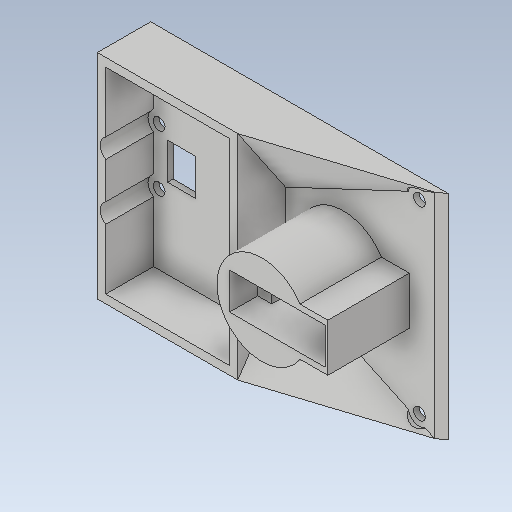
# Autodesk Inventor part: cover
Saved by Autodesk Inventor 2020 (Build 240168000, 168)
## iProperties
Created: 2020-01-29
Part Number: cover
Material: Ogólne
Document SubType Name: Modeling
Designer: blep
Density: 1 g/cm^3
Appearance: Domyślne
Author: blep
Autodesk Inventor part; units mm, degrees
ref_plane "YZ Plane" through (0, 0, 0) normal (1, 0, 0) x (0, 1, 0)
ref_plane "XZ Plane" through (0, 0, 0) normal (0, 1, 0) x (-1, 0, 0)
ref_plane "XY Plane" through (0, 0, 0) normal (0, 0, 1) x (1, 0, 0)
sketch "Sketch1" plane through (0, 0, 0) normal (0, 0, 1) x (1, 0, 0)
  line L0 (47.7059, -35) -> (-50, -35) projected
  line L1 (-50, -35) -> (-50, 35) projected
  line L2 (-50, 35) -> (47.7059, 35) projected
  line L3 (47.7059, 35) -> (47.7059, -35) projected
  line L4 (53, -38) -> (53, 38) projected
  line L5 (53, 38) -> (-53, 38) projected
  line L6 (-53, 38) -> (-53, -38) projected
  line L7 (-53, -38) -> (53, -38) projected
  point P0 (0, 0)
extrude "Extrusion1" add sketch "Sketch1" along normal blind 2 contours L0 L1 L2 L3 | L7 L6 L5 L4
sketch "Sketch2" plane through (-53, 38, 0) normal (0, 1, 0) x (1, 0, 0)
  line L0 (106, 0) -> (130.7184, 17) projected
  line L1 (106, 0) -> (106, -2) projected
  line L2 (106, 0) -> (103.092, -2)
  line L3 (106, -2) -> (0, -2) projected
  line L4 (103.092, -2) -> (106, -2)
  point P0 (53, 0)
  constraints: 4 end point, 1 collinear, 1 point on line
extrude "Extrusion2" cut sketch "Sketch2" against normal through all
sketch "Sketch3" plane through (0, 0, 2) normal (0, 0, 1) x (1, 0, 0)
  line L0 (50.092, -38) -> (50.092, 38) projected
  line L1 (50.092, 38) -> (-53, 38) projected
  line L2 (-53, 38) -> (-53, -38) projected
  line L3 (-53, -38) -> (50.092, -38) projected
  line L4 (-53, -38) -> (-3, -38)
  line L5 (-3, -38) -> (-3, 38)
  line L6 (-3, 38) -> (-53, 38)
  line L7 (-53, 38) -> (-53, -38)
  line L8 (-53, 38) -> (-53, -38) projected
  line L9 (-53, -38) -> (50.092, -38) projected
  line L10 (50.092, 38) -> (-53, 38) projected
  line L11 (-50, -35) -> (-6, -35)
  line L12 (-6, -35) -> (-6, 35)
  line L13 (-6, 35) -> (-50, 35)
  line L14 (-50, 35) -> (-50, -35)
  point P0 (0, 0)
  dimension "d4" = 50
  dimension "d5" = 3
  dimension "d6" = 3
  dimension "d7" = 3
  dimension "d8" = 3
  constraints: 16 end point, 4 parallel, 3 collinear, 2 horizontal, 2 perpendicular
  measures "d4" distance between parallel lines of L2 L5
  measures "d5" distance between parallel lines of L2 L14
  measures "d6" distance between parallel lines of L3 L11
  measures "d7" distance between parallel lines of L1 L13
  measures "d8" distance between parallel lines of L5 L12
extrude "Extrusion3" add sketch "Sketch3" along normal blind 17 contours L3 L2 L1 L5
sketch3d "3D Sketch1"
sketch "Sketch4" plane through (-3, -38, 2) normal (1, 0, 0) x (0, 0, -1)
  line L0 (0, 76) -> (0, 0) projected
  line L1 (0, 76) -> (-17, 76) projected
  line L2 (-17, 0) -> (-17, 76) projected
  line L3 (0, 0) -> (-17, 0) projected
  line L4 (-17, 0) -> (-17, 76) projected
  line L5 (-17, 0) -> (0, 25)
  line L6 (0, 3) -> (0, 73) projected
  line L7 (-17, 76) -> (0, 51)
  point P0 (2, 38)
  dimension "d11" = 25
  dimension "d12" = 25
  constraints: 4 end point, 2 point on line
  measures "d11" distance from line of L3 L5.end
  measures "d12" distance from line of L1 L7.end
loft "Loft1" add profiles "Sketch4" section 2 point at (50.092, -38, 2) contours L5 L0 L3
loft "Loft2" add profiles "Sketch4" section 2 point at (50.092, 38, 2) contours L0 L7 L1
sketch "Sketch6" plane through (0, 0, 2) normal (0, 0, 1) x (1, 0, 0)
  line L0 (11.092, -6.5) -> (35.092, -6.5)
  line L1 (35.092, -6.5) -> (35.092, 6.5)
  line L2 (35.092, 6.5) -> (11.092, 6.5)
  line L3 (11.092, 6.5) -> (11.092, -6.5)
  line L4 (50.092, -38) -> (50.092, 38) construction
  line L5 (50.092, 38) -> (35.092, 6.5) construction
  line L6 (50.092, -38) -> (35.092, -6.5) construction
  line L7 (11.092, -6.5) -> (35.092, 6.5) construction
  line L8 (11.092, 6.5) -> (35.092, -6.5) construction
  line L9 (5.092, -8.5) -> (41.092, -8.5)
  line L10 (41.092, -8.5) -> (41.092, 8.5)
  line L11 (41.092, 8.5) -> (5.092, 8.5)
  line L12 (5.092, 8.5) -> (5.092, -8.5)
  point P0 (0, 0)
  point P1 (23.092, 0)
  dimension "d25" = 24
  dimension "d26" = 13
  dimension "d27" = 15
  dimension "d31" = 6
  dimension "d32" = 6
  dimension "d33" = 2
  dimension "d34" = 2
  constraints: 24 end point, 4 parallel, 2 horizontal, 2 perpendicular, 1 equal length, 1 midpoint
  measures "d25" distance of L2.end L1.end
  measures "d26" distance of L1.end L0.end
  measures "d27" distance between parallel lines of L4 L1
  measures "d31" distance between parallel lines of L12 L3
  measures "d32" distance between parallel lines of L10 L1
  measures "d33" distance between parallel lines of L9 L0
  measures "d34" distance between parallel lines of L11 L2
extrude "Extrusion5" add sketch "Sketch6" along normal blind 19
sketch "Sketch7" plane through (0, 0, 2) normal (0, 0, 1) x (1, 0, 0)
  circle A0 centre (17.592, 0) radius 0.6 projected
  arc A1 (31.1474, 8.5) -> (31.1474, -8.5) centre (17.592, 0) ccw
  line L0 (31.1474, -8.5) -> (5.092, -8.5)
  line L1 (5.092, -8.5) -> (5.092, 8.5)
  line L2 (5.092, 8.5) -> (31.1474, 8.5)
  line L3 (5.092, -8.5) -> (5.092, 8.5) projected
  line L4 (41.092, -8.5) -> (5.092, -8.5) projected
  line L5 (5.092, 8.5) -> (41.092, 8.5) projected
  point P0 (0, 0)
  dimension "d35" = 32
  constraints: 6 end point, 3 collinear, 2 point on circle, 2 point on line, 1 centre point, 1 coincident
  measures "d35" diameter of A1
extrude "Extrusion6" add sketch "Sketch7" along normal blind 19 contours L2 L1 L0 A1
sketch "Sketch8" plane through (0, 0, 21) normal (0, 0, 1) x (1, 0, 0)
  line L0 (6.592, -1.125) -> (6.592, -6.2) projected
  line L1 (6.592, 6.2) -> (6.592, 1.125) projected
  line L2 (11.092, 6.5) -> (35.092, 6.5) projected
  line L3 (35.092, -6.5) -> (11.092, -6.5) projected
  line L4 (39.592, 6.2) -> (39.592, 1.125) projected
  line L5 (39.592, -1.125) -> (39.592, -6.2) projected
  line L6 (6.092, -6.5) -> (40.092, -6.5)
  line L7 (40.092, -6.5) -> (40.092, 6.5)
  line L8 (40.092, 6.5) -> (6.092, 6.5)
  line L9 (6.092, 6.5) -> (6.092, -6.5)
  arc A0 (31.1474, 8.5) -> (31.1474, -8.5) centre (17.592, 0) ccw projected
  line L10 (31.1474, -8.5) -> (41.092, -8.5) projected
  line L11 (41.092, 8.5) -> (31.1474, 8.5) projected
  line L12 (41.092, -8.5) -> (41.092, 8.5) projected
  point P0 (0, 0)
  dimension "d38" = 0.5
  dimension "d39" = 0.5
  constraints: 8 end point, 2 collinear, 2 parallel, 1 horizontal, 1 perpendicular
  measures "d38" distance between parallel lines of L7 L4
  measures "d39" distance between parallel lines of L1 L9
ref_plane "Work Plane1" through (12.092, -5.5, 31) normal (0, 0, 1) x (1, 0, 0)
extrude "Extrusion7" add sketch "Sketch8" along normal up to surface (10 mm away)
sketch "Sketch9" plane through (0, 0, 21) normal (0, 0, 1) x (1, 0, 0)
  arc A0 (8.4305, -0.75) -> (8.4305, 0.75) centre (9.092, 0) ccw projected
  arc A1 (37.7534, 0.75) -> (37.7534, -0.75) centre (37.092, 0) ccw projected
  point P0 (0, 0)
hole "Hole1" at (9.092, 0, 21) at (37.092, 0, 21) direction (0, 0, -1) diameter 1 depth 5 tip angle 118
sketch "Sketch10" plane through (0, 0, 2) normal (0, 0, 1) x (1, 0, 0)
  line L0 (7.592, -4.5) -> (11.092, -4.5)
  line L1 (11.092, -4.5) -> (11.092, 4.5)
  line L2 (11.092, 4.5) -> (7.592, 4.5)
  line L3 (7.592, 4.5) -> (7.592, -4.5)
  line L4 (11.092, 6.5) -> (11.092, -6.5) projected
  line L5 (35.092, 6.5) -> (11.092, 6.5) construction
  line L6 (11.092, 6.5) -> (7.592, 4.5) construction
  line L7 (7.592, -4.5) -> (11.092, -6.5) construction
  point P0 (0, 0)
  dimension "d49" = 3.5
  dimension "d50" = 9
  constraints: 12 end point, 2 parallel, 1 collinear, 1 equal length, 1 horizontal, 1 perpendicular
  measures "d49" distance of L2.end L1.end
  measures "d50" distance of L1.end L0.end
extrude "Extrusion8" cut sketch "Sketch10" along normal blind 14 and the other way blind 3
sketch "Sketch11" plane through (0, 0, 0) normal (0, 0, -1) x (-1, 0, 0)
  circle A0 centre (-44.7059, -33) radius 2.125 projected
  circle A1 centre (-44.7059, 33) radius 2.125 projected
  circle A2 centre (48, -10) radius 2.125 projected
  circle A3 centre (48, 10) radius 2.125 projected
  point P0 (0, 0)
extrude "Extrusion9" cut sketch "Sketch11" against normal through all
sketch "Sketch12" plane through (0, 0, 2) normal (0, 0, 1) x (1, 0, 0)
  circle A0 centre (44.7059, -33) radius 2.125 projected
  circle A1 centre (44.7059, 33) radius 2.125 projected
  arc A2 (-50, -10.7181) -> (-50, -9.2819) centre (-48, -10) ccw projected
  arc A3 (-50, 9.2819) -> (-50, 10.7181) centre (-48, 10) ccw projected
  circle A4 centre (44.7059, -33) radius 4
  circle A5 centre (44.7059, 33) radius 4
  circle A6 centre (-48, -10) radius 2.125 projected
  circle A7 centre (-48, -10) radius 4
  circle A8 centre (-48, 10) radius 2.125 projected
  circle A9 centre (-48, 10) radius 4
  point P0 (0, 0)
  dimension "d57" = 8
  dimension "d58" = 8
  dimension "d59" = 8
  dimension "d60" = 8
  constraints: 4 centre point, 4 coincident
  measures "d57" diameter of A4
  measures "d58" diameter of A5
  measures "d59" diameter of A7
  measures "d60" diameter of A9
extrude "Extrusion10" cut sketch "Sketch12" along normal through all contours A0 | A1 | A6 A2 | A8 A3 | A4 | A5 | A7 | A9
sketch "Sketch15" plane through (0, 0, 2) normal (0, 0, 1) x (1, 0, 0)
  line L0 (-45, -6.5) -> (-35, -6.5)
  line L1 (-35, -6.5) -> (-35, 6.5)
  line L2 (-35, 6.5) -> (-45, 6.5)
  line L3 (-45, 6.5) -> (-45, -6.5)
  line L4 (-50, -35) -> (-50, -13.4641) construction
  line L5 (-50, -35) -> (-45, -6.5) construction
  line L6 (-50, 35) -> (-6, 35) construction
  line L7 (-45, 6.5) -> (-50, 35) construction
  line L8 (-50, -6.5359) -> (-50, 6.5359) construction
  circle A0 centre (11, -17) radius 2
  line L9 (-3, -38) -> (-3, 38) projected
  line L10 (-3, -38) -> (50.092, -38) projected
  point P0 (0, 0)
  dimension "d73" = 10
  dimension "d74" = 13
  dimension "d75" = 5
  dimension "d76" = 4
  dimension "d77" = 14
  dimension "d78" = 21
  constraints: 12 end point, 2 parallel, 1 centre point, 1 equal length, 1 horizontal, 1 perpendicular
  measures "d73" distance of L2.end L1.end
  measures "d74" distance of L1.end L0.end
  measures "d75" distance between parallel lines of L8 L3
  measures "d76" diameter of A0
  measures "d77" distance from line of L9 A0.centre
  measures "d78" distance from line of L10 A0.centre
extrude "Extrusion12" cut sketch "Sketch15" against normal through all
equation "\"d6\" = d5"
equation "\"d7\" = d5"
equation "\"d8\" = d5"
equation "\"d12\" = d11"
equation "\"d32\" = d31"
equation "\"d34\" = d33"
equation "\"d39\" = d38"
body "Solid1"
